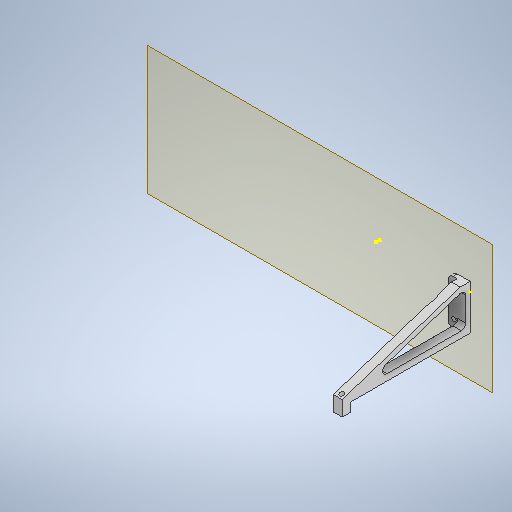
# Autodesk Inventor part: wzmocnienie
Saved by Autodesk Inventor 2025.1 (Build 291241000, 241)
## iProperties
Created: 2024-11-04
Part Number: wzmocnienie
Material: Ogólny
Document SubType Name: Modeling
Designer: PC
Density: 1 g/cm^3
Appearance: Domyślna
Author: PC
Autodesk Inventor part; units mm, degrees
ref_plane "YZ Plane" through (0, 0, 0) normal (1, 0, 0) x (0, 1, 0)
ref_plane "XZ Plane" through (0, 0, 0) normal (0, 1, 0) x (-1, 0, 0)
ref_plane "XY Plane" through (0, 0, 0) normal (0, 0, 1) x (1, 0, 0)
ref_plane "Płaszczyzna konstrukcyjna2" through (0, 0, 0) normal (0, 0, 1) x (1, 0, 0)
sketch "Szkic2" plane through (0, 0, 0) normal (0, 0, 1) x (1, 0, 0)
  circle A0 centre (53.2, -19.05) radius 2 projected
  circle A1 centre (53.2, 1.9) radius 2 projected
  line L0 (61.2, -24.6614) -> (49.2, -24.6614)
  line L1 (49.2, -24.6614) -> (49.2, 5.9)
  line L2 (49.2, 5.9) -> (61.2, 5.9)
  line L3 (61.2, 5.9) -> (61.2, -24.6614)
  line L4 (60, -30.65) -> (57, -30.65) projected
  point P0 (0, 0)
  dimension "d0" = 4
  dimension "d1" = 4
  dimension "d2" = 12
  dimension "d3" = 30.5614
  constraints: 8 end point, 2 parallel, 1 horizontal, 1 perpendicular
  measures "d0" distance from line of L2 A1.centre
  measures "d1" distance from line of L1 A1.centre
  measures "d2" distance between parallel lines of L1 L3
  measures "d3" distance of L2.end L0.start
extrude "Wyciągnięcie proste1" add sketch "Szkic2" along normal blind 87.3125 contours A0 | A1 | L0 L1 L2 L3
sketch "Szkic3" plane through (49.2, -24.6614, 0) normal (0, -1, 0) x (1, 0, 0)
  circle A0 centre (9.3, 84.9) radius 1.5 projected
  circle A1 centre (9.3, 84.9) radius 1.45
  point P0 (-49.2, 0)
  dimension "d6" = 2.9
  constraints: 1 centre point, 1 coincident
  measures "d6" diameter of A1
extrude "Wyciągnięcie proste2" cut sketch "Szkic3" against normal blind 10 contours A1
sketch "Szkic4" plane through (0, 0, 0) normal (0, 0, -1) x (-1, 0, 0)
  point P0 (0, 0)
sketch "Szkic6" plane through (61.2, -24.6614, 0) normal (1, 0, 0) x (0, 0, -1)
  point P0 (0, 24.6614)
sketch "Szkic5" plane through (0, 0, 0) normal (0, 0, -1) x (-1, 0, 0)
  circle A0 centre (-53.2, 1.9) radius 2 projected
  circle A1 centre (-53.2, -19.05) radius 2 projected
  circle A2 centre (-53.2, -19.05) radius 1.45
  circle A3 centre (-53.2, 1.9) radius 1.45
  point P0 (0, 0)
  dimension "d9" = 2.9
  dimension "d10" = 2.9
  constraints: 2 centre point, 2 coincident
  measures "d9" diameter of A2
  measures "d10" diameter of A3
extrude "Wyciągnięcie proste3" cut sketch "Szkic5" against normal blind 6 contours A2 | A3
sketch "Szkic7" plane through (61.2, -24.6614, 0) normal (1, 0, 0) x (0, 0, -1)
  line L0 (-87.3125, 30.5614) -> (-87.3125, 0) projected
  line L1 (-87.3125, 4.3495) -> (-6.8101, 30.5614)
  line L2 (-57.6962, 10.2021) -> (-6.9288, 26.7322)
  line L3 (0, 28.0114) -> (-6, 28.0114) projected
  line L4 (-3, 23.8796) -> (-3, 7.3495)
  line L5 (-6, 4.3495) -> (-56.7674, 4.3495)
  line L6 (0, 30.5614) -> (-87.3125, 30.5614) projected
  arc A0 (-57.6962, 10.2021) -> (-56.7674, 4.3495) centre (-56.7674, 7.3495) ccw
  arc A1 (-6, 4.3495) -> (-3, 7.3495) centre (-6, 7.3495) ccw
  arc A2 (-3, 23.8796) -> (-6.9288, 26.7322) centre (-6, 23.8796) ccw
  point P0 (0, 24.6614)
  point P1 (-75.6708, 4.3495)
  point P2 (-3, 28.0114)
  point P3 (-3, 4.3495)
  dimension "d17" = 3
  constraints: 8 end point, 8 point on line, 6 point on circle, 6 tangent, 3 centre point, 2 equal radius, 1 midpoint, 1 parallel, 1 perpendicular, 1 vertical
  measures "d17" radius of A0
extrude "Wyciągnięcie proste4" cut sketch "Szkic7" against normal blind 14.7625
sketch "Szkic8" plane through (49.2, -24.6614, 0) normal (0, -1, 0) x (1, 0, 0)
  line L0 (0, 87.3125) -> (12, 87.3125) projected
  line L1 (0, 0) -> (0, 6.8101) projected
  line L2 (12, 0) -> (12, 87.3125) projected
  line L3 (0, 0) -> (0, 87.3125) projected
  line L4 (0, 0) -> (12, 0) projected
  line L5 (6, 87.3125) -> (6, 3)
  line L6 (12, 3) -> (0, 3) projected
  point P0 (-49.2, 0)
  constraints: 2 end point, 2 midpoint, 1 vertical
extrude "Wyciągnięcie proste5" cut sketch "Szkic8" against normal blind 30.6375 contours L0 L5 L6 L1 L3
sketch "Szkic9" plane through (49.2, -24.6614, 0) normal (0, -1, 0) x (1, 0, 0)
  line L0 (6, 87.3125) -> (6, 3) projected
  line L1 (12, 6.8101) -> (12, 87.3125) projected
  line L2 (6, 87.3125) -> (12, 87.3125)
  line L3 (12, 87.3125) -> (12, 81.8248)
  line L4 (12, 81.8248) -> (6, 81.8248)
  line L5 (6, 81.8248) -> (6, 87.3125)
  circle A0 centre (9.3, 84.9) radius 1.5 projected
  point P0 (-49.2, 0)
  constraints: 8 end point, 2 parallel, 1 horizontal, 1 perpendicular, 1 point on line
ref_plane "Płaszczyzna konstrukcyjna3" through (-147.5, -30.65, -16.2) normal (0, 1, 0) x (0, 0, 1)
extrude "Wyciągnięcie proste6" add sketch "Szkic9" along normal up to surface (5.9886 mm away)
sketch "Szkic10" plane through (61.2, -17.3119, 3) normal (0, 0, 1) x (1, 0, 0)
  point P0 (-61.2, 17.3119)
sketch "Szkic11" plane through (61.2, -17.3119, 3) normal (0, 0, 1) x (1, 0, 0)
  circle A0 centre (-8, -1.7381) radius 1.45 projected
  circle A1 centre (-8, 19.2119) radius 1.45 projected
  circle A2 centre (-8, -1.7381) radius 1.45 projected
  circle A3 centre (-8, -1.7381) radius 2.5
  circle A4 centre (-8, 19.2119) radius 2.5
  point P0 (-61.2, 17.3119)
  dimension "d20" = 5
  constraints: 2 centre point, 2 coincident, 1 equal radius
  measures "d20" diameter of A3
extrude "Wyciągnięcie proste7" cut sketch "Szkic11" along normal blind 28.575 contours A0 | A1 | A3 | A4
fillet "Zaokrąglenie1" radius 3.175 2 edges at (49.2, 5.9, 1.5) (49.2, -24.6614, 1.5)
